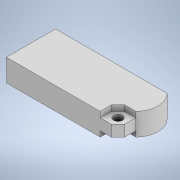
# Autodesk Inventor part: Prototype
Saved by Autodesk Inventor 2020 (Build 240168000, 168)
## iProperties
Created: 2022-05-09
Part Number: Prototype
Material: Типовые
Document SubType Name: Modeling
Designer: NoName
Density: 1 g/cm^3
Appearance: По умолчанию
Author: NoName
Autodesk Inventor part; units mm, degrees
ref_plane "YZ Plane" through (0, 0, 0) normal (1, 0, 0) x (0, 1, 0)
ref_plane "XZ Plane" through (0, 0, 0) normal (0, 1, 0) x (-1, 0, 0)
sketch "Эскиз1" plane through (0, 0, 0) normal (0, 1, 0) x (-1, 0, 0)
  line L0 (0, -11) -> (-50, -11)
  arc A0 (-50, 3) -> (-50, -11) centre (-42.8586, -4) ccw
  line L1 (-42, 11) -> (0, 11)
  line L2 (-50, 3) -> (-45, 3)
  line L3 (-45, 3) -> (-42, 6)
  line L4 (-42, 6) -> (-42, 11)
  line L5 (0, -11) -> (0, 11)
  point P0 (0, 0)
  point P1 (0, 0)
  dimension "d3" = 50
  dimension "d4" = 7
  dimension "d5" = 10
  dimension "d9" = 45
  dimension "d10" = 3
  dimension "d11" = 22
  constraints: 12 end point, 3 horizontal, 2 perpendicular, 2 point on circle, 1 centre point, 1 coincident, 1 midpoint, 1 vertical, 1 vertical alignment
  measures "d3" distance of L0.start L0.end
  measures "d4" distance from line of L0 A0.centre
  measures "d5" radius of A0
  measures "d9" angle of L2 L3
  measures "d10" horizontal distance of L2.end L3.end
  measures "d11" distance of L0.start L1.end
extrude "Выдавливание1" add sketch "Эскиз1" along normal blind 10
ref_plane "РабПлоскость1" through (0, 5, 0) normal (0, 1, 0) x (1, 0, 0)
sketch "Эскиз6" plane through (0, 5, 0) normal (0, 1, 0) x (1, 0, 0)
  line L0 (50, 11) -> (0, 11) projected
  line L1 (0, 11) -> (0, -11) projected
  line L2 (0, -11) -> (42, -11) projected
  line L3 (42, -11) -> (42, -6) projected
  line L4 (42, -6) -> (45, -3) projected
  line L5 (45, -3) -> (50, -3) projected
  arc A0 (50, -3) -> (50, 11) centre (42.8586, 4) ccw projected
  line L6 (45, -3) -> (50, -3) projected
  line L7 (50, -3) -> (50, -8)
  line L8 (50, -8) -> (47, -11)
  line L9 (0, -11) -> (42, -11) projected
  line L10 (47, -11) -> (42, -11)
  line L11 (42, -6) -> (45, -3) projected
  arc A1 (50, -3) -> (50, 11) centre (42.8586, 4) ccw projected
  line L12 (42, -11) -> (50, -3) construction
  circle A2 centre (46, -7) radius 2
  point P0 (0, 0)
  dimension "d25" = 4
  constraints: 8 end point, 2 parallel, 1 centre point, 1 collinear, 1 midpoint, 1 vertical
  measures "d25" diameter of A2
extrude "Выдавливание4" add sketch "Эскиз6" along normal mid plane 5 contours L7 L8 L10 L3 L4 L5
